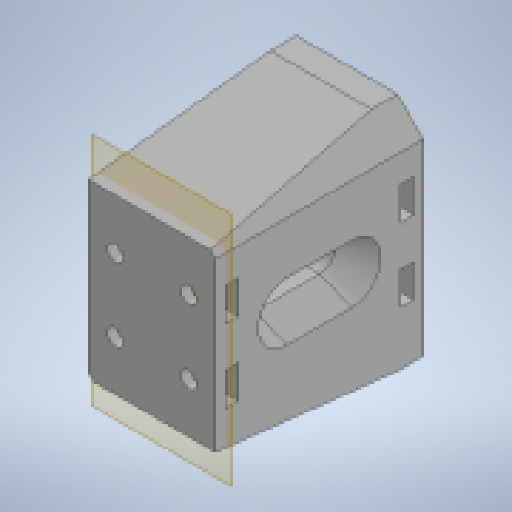
# Autodesk Inventor part: MCP-IV
Saved by Autodesk Inventor 2026 (Build 300175050, 175E)
## iProperties
Created: 2025-12-08
Part Number: MCP-IV
Material: Genérico
Document SubType Name: Modeling
Designer: user
Density: 1 g/cm^3
Appearance: Gris claro
Author: user
Autodesk Inventor part; units mm, degrees
ref_plane "YZ Plane" through (0, 0, 0) normal (1, 0, 0) x (0, 1, 0)
ref_plane "XZ Plane" through (0, 0, 0) normal (0, 1, 0) x (-1, 0, 0)
ref_plane "Plano de trabajo1" through (-9.8, -13.3, 23.9585) normal (0, 0, -1) x (0, 1, 0)
sketch "Boceto1" plane through (0, 0, 0) normal (0, 0, 1) x (1, 0, 0)
  line L0 (9.8, 13.3) -> (9.8, -13.3) projected
  line L1 (-9.8, -13.3) -> (9.8, -13.3) projected
  line L2 (-9.8, -13.3) -> (-9.8, 13.3) projected
  line L3 (9.8, 13.3) -> (-9.8, 13.3) projected
  circle A0 centre (8, 8) radius 0.8 projected
  circle A1 centre (-8, -8) radius 0.8 projected
  circle A2 centre (8, -8) radius 0.8 projected
  circle A3 centre (0, 0) radius 4 projected
  circle A4 centre (0, 6) radius 1.025 projected
  circle A5 centre (6, 0) radius 1.025 projected
  circle A6 centre (0, -6) radius 1.025 projected
  circle A7 centre (-6, 0) radius 1.025 projected
  circle A8 centre (5.6569, 5.6569) radius 1.025 projected
  circle A9 centre (5.6569, -5.6569) radius 1.025 projected
  circle A10 centre (-5.6569, -5.6569) radius 1.025 projected
  circle A11 centre (-5.6569, 5.6569) radius 1.025 projected
  circle A12 centre (-3, 9) radius 1.025 projected
  circle A13 centre (3, 9) radius 1.025 projected
  circle A14 centre (-3, -9) radius 1.025 projected
  circle A15 centre (3, -9) radius 1.025 projected
  circle A16 centre (-8, 8) radius 0.8 projected
  circle A17 centre (-5.6569, -5.6569) radius 1.25
  circle A18 centre (-5.6569, 5.6569) radius 1.25
  circle A19 centre (5.6569, 5.6569) radius 1.25
  circle A20 centre (5.6569, -5.6569) radius 1.25
  line L4 (9.7, -16.5) -> (-9.7, -16.5) projected
  line L5 (9.7, 16.5) -> (-9.7, 16.5) projected
  line L6 (-9.8, 13.3) -> (9.8, 13.3)
  line L7 (9.8, 13.3) -> (9.8, -16.5)
  line L8 (9.8, -16.5) -> (-9.8, -16.5)
  line L9 (-9.8, -16.5) -> (-9.8, 13.3)
  line L10 (-9.8, -13.3) -> (9.8, -13.3)
  line L11 (9.8, -13.3) -> (9.8, 16.5)
  line L12 (9.8, 16.5) -> (-9.8, 16.5)
  line L13 (-9.8, 16.5) -> (-9.8, -13.3)
  point P0 (0, 0)
  point P1 (9.8, 13.3)
  dimension "d30" = 2.5
  constraints: 16 end point, 4 centre point, 4 collinear, 4 parallel, 3 equal radius, 2 horizontal, 2 perpendicular
  measures "d30" diameter of A17
extrude "Extrusión1" add sketch "Boceto1" along normal blind 16.0175 contours L0 L1 L2 L3 | L3 L13 L12 L5 L11 | L7 L8 L4 L9 L1 | A0 | A1 | A2 | A3 | A4 | A5 | A6 | A7 | A12 | A13 | A14 | A15 | A16
ref_plane "Plano de trabajo2" through (0, 0, 14.5175) normal (0, 0, 1) x (1, 0, 0)
sketch "Boceto2" plane through (0, 0, 14.5175) normal (0, 0, -1) x (-1, 0, 0)
  line L0 (-7.6569, -4.5022) -> (-5.6569, -3.3475) construction
  line L1 (-5.6569, -3.3475) -> (-3.6569, -4.5022) construction
  line L2 (-3.6569, -4.5022) -> (-3.6569, -6.8116) construction
  line L3 (-3.6569, -6.8116) -> (-5.6569, -7.9663) construction
  line L4 (-5.6569, -7.9663) -> (-7.6569, -6.8116) construction
  line L5 (-7.6569, -6.8116) -> (-7.6569, -4.5022) construction
  line L6 (-5.6569, -3.1165) -> (-7.8569, -4.3867)
  line L7 (-7.8569, -4.3867) -> (-7.8569, -6.927)
  line L8 (-7.8569, -6.927) -> (-5.6569, -8.1972)
  line L9 (-5.6569, -8.1972) -> (-3.4569, -6.927)
  line L10 (-3.4569, -6.927) -> (-3.4569, -4.3867)
  line L11 (-3.4569, -4.3867) -> (-5.6569, -3.1165)
  line L12 (-5.6569, -8.1972) -> (-9.8, -8.1972)
  line L13 (-5.6569, -3.1165) -> (-9.8, -3.1165)
  line L14 (0, -13.7812) -> (0, 16.5) construction
  line L15 (-10.9793, 0) -> (10.9793, 0) construction
  line L16 (-5.6569, 3.1165) -> (-7.8569, 4.3867)
  line L17 (-7.8569, 4.3867) -> (-7.8569, 6.927)
  line L18 (-7.8569, 6.927) -> (-5.6569, 8.1972)
  line L19 (-5.6569, 8.1972) -> (-3.4569, 6.927)
  line L20 (-3.4569, 6.927) -> (-3.4569, 4.3867)
  line L21 (-3.4569, 4.3867) -> (-5.6569, 3.1165)
  line L22 (-5.6569, 8.1972) -> (-9.8, 8.1972)
  line L23 (-5.6569, 3.1165) -> (-9.8, 3.1165)
  line L24 (5.6569, -3.1165) -> (7.8569, -4.3867)
  line L25 (7.8569, -4.3867) -> (7.8569, -6.927)
  line L26 (7.8569, -6.927) -> (5.6569, -8.1972)
  line L27 (5.6569, -8.1972) -> (3.4569, -6.927)
  line L28 (3.4569, -6.927) -> (3.4569, -4.3867)
  line L29 (3.4569, -4.3867) -> (5.6569, -3.1165)
  line L30 (5.6569, -8.1972) -> (9.8, -8.1972)
  line L31 (5.6569, -3.1165) -> (9.8, -3.1165)
  line L32 (5.6569, 8.1972) -> (3.4569, 6.927)
  line L33 (3.4569, 6.927) -> (3.4569, 4.3867)
  line L34 (3.4569, 4.3867) -> (5.6569, 3.1165)
  line L35 (5.6569, 3.1165) -> (9.8, 3.1165)
  line L36 (5.6569, 3.1165) -> (7.8569, 4.3867)
  line L37 (7.8569, 4.3867) -> (7.8569, 6.927)
  line L38 (7.8569, 6.927) -> (5.6569, 8.1972)
  line L39 (5.6569, 8.1972) -> (9.8, 8.1972)
  circle A0 centre (-5.6569, -5.6569) radius 1.25 construction
  circle A1 centre (-5.6569, 5.6569) radius 1.25 construction
  circle A2 centre (5.6569, 5.6569) radius 1.25 construction
  circle A3 centre (5.6569, -5.6569) radius 1.25 construction
  line L40 (9.8, 16.5) -> (-9.8, 16.5) projected
  line L41 (-9.8, 16.5) -> (-9.8, -16.5) projected
  line L42 (-9.8, -16.5) -> (9.8, -16.5) projected
  line L43 (9.8, -16.5) -> (9.8, 16.5) projected
  point P0 (0, 0)
  point P1 (0, 0)
  dimension "d3" = 4.6188
  dimension "d102" = 0.2
  constraints: 80 end point, 24 symmetric about line, 3 horizontal, 2 midpoint, 2 point on line, 2 vertical, 1 coincident, 23 other
  measures "d3" distance of L0.end L3.end
  measures "d102" distance between parallel lines of L0 L6
extrude "Extrusión2" cut sketch "Boceto2" along normal blind 2 contours L11 L10 L9 L8 L7 L6 | L6 L7 L8 L12 L41 L13 | L41 L22 L18 L17 L16 L23 | L16 L17 L18 L19 L20 L21 | L30 L26 L25 L24 L31 L43 | L43 L35 L36 L37 L38 L39 | L27 L28 L29 L24 L25 L26 | L38 L37 L36 L34 L33 L32
mirror "Simetría2" about plane through (0, 0, 0) normal (0, 0, 1)
sketch "Boceto4" plane through (0, 0, 16.0175) normal (0, 0, 1) x (1, 0, 0)
  line L0 (9.8, -16.5) -> (9.8, 16.5) projected
  line L1 (-9.8, 16.5) -> (-9.8, -16.5) projected
  circle A0 centre (5.6569, 5.6569) radius 1.25 construction
  circle A1 centre (-5.6569, -5.6569) radius 1.25 construction
  circle A2 centre (-5.6569, -5.6569) radius 2.3094 construction
  circle A3 centre (-5.6569, -5.6569) radius 2.8094
  circle A4 centre (5.6569, 5.6569) radius 2.8094
  line L2 (-9.8, -16.5) -> (9.8, -16.5) projected
  line L3 (9.8, 16.5) -> (-9.8, 16.5) projected
  point P0 (0, 0)
  point P1 (-5.6569, -7.9663)
  point P2 (-7.6569, -4.5022)
  point P3 (-3.6569, -4.5022)
  dimension "d81" = 1.3337
  dimension "d84" = 360
  dimension "d91" = 0.5
  dimension "d92" = 5.6188
  constraints: 3 centre point, 3 point on circle, 5 other
  measures "d81" distance edge to line of A3 L1
  measures "d91" radial gap between concentric circles of A3 A2
  measures "d92" diameter of A3
extrude "Extrusión3" [suppressed]
chamfer "Chaflán1" [suppressed]
chamfer "Chaflán4" [suppressed]
pattern_circular "Patrón circular1" [suppressed]
chamfer "Chaflán2" distance 3.2 distance2 28.035 2 edges at (0, -16.5, 16.0175) (0, 16.5, 16.0175) measured on face at (1.6489, 13.2285, 16.0175)
chamfer "Chaflán6" distance 4 angle 45 8 edges at (-9.8, -16.5, -14.0175) (9.8, 16.5, -14.0175) (-9.8, 14.9, 2) (-9.8, 16.5, -14.0175) (9.8, -14.9, 2) (9.8, -16.5, -14.0175) (9.8, 14.9, 2) (-9.8, -14.9, 2)
sketch "Boceto5" plane through (0, 0, 0) normal (1, 0, 0) x (0, 1, 0)
  line L0 (0, 0) -> (0, 15.987) construction
  line L1 (0, -5) -> (0, 5) construction
  line L2 (2.5, -5) -> (2.5, 5)
  line L3 (-2.5, 5) -> (-2.5, -5)
  arc A0 (-2.5, -5) -> (2.5, -5) centre (0, -5) ccw
  arc A1 (2.5, 5) -> (-2.5, 5) centre (0, 5) ccw
  dimension "d93" = 5
  dimension "d100" = 15
  constraints: 10 end point, 4 point on circle, 4 tangent, 2 centre point, 1 midpoint, 1 parallel, 1 point on line, 1 vertical
  measures "d93" diameter of A1
extrude "Extrusión4" cut sketch "Boceto5" along normal through all both and the other way through all
chamfer "Chaflán5" distance 2 distance2 5 4 edges at (-9.8, 0, 7.5) (-9.8, -2.5, 0) (-9.8, 0, -7.5) (-9.8, 2.5, 0) measured on face at (-9.8, 7.7324, 1.7575)
chamfer "Chaflán7" distance 2 distance2 5 4 edges at (9.8, 0, 7.5) (9.8, 2.5, 0) (9.8, 0, -7.5) (9.8, -2.5, 0) measured on face at (9.8, -7.7324, 1.7575)
equation "\"d3\" = d2"
equation "\"d2\" = 4.618802"
